gear-pinion-9 v1 (Autodesk Fusion 360 design; units mm, degrees)
description: Spur Gear; Module: 0.3; Num Teeth: 9; Pressure Angle: 20.0; Backlash: 0.00 mm
Autodesk Fusion 360 part; units mm, degrees
sketch "スケッチ1" plane through (0, 0, 0) normal (0, 0, 1) x (1, 0, 0) in component "Spur Gear (9 teeth)"
  circle A0 centre (0, 0) radius 0.9392
  circle A1 centre (0, 0) radius 0.4
extrude "押し出し1" add sketch "スケッチ1" along normal blind 1 in component "Spur Gear (9 teeth)"
sketch "スケッチ2" plane through (0, 0, 0) normal (0, 0, 1) x (1, 0, 0) in component "Spur Gear (9 teeth)"
  spline S0 degree 5 poles (1.2459, -0.2389) (1.247, -0.2391) (1.2492, -0.2395) (1.2525, -0.2399) (1.2569, -0.2403) (1.2625, -0.2405) (1.268, -0.2404) (1.2736, -0.2403) (1.2793, -0.24) (1.2849, -0.2397) (1.2906, -0.2394) (1.2962, -0.2389) (1.3019, -0.2384) (1.3076, -0.2378) (1.3134, -0.237) (1.3191, -0.2362) (1.3248, -0.2353) (1.3306, -0.2342) (1.3363, -0.2332) (1.3421, -0.232) (1.3478, -0.2308) (1.3536, -0.2295) (1.3594, -0.2282) (1.3652, -0.2268) (1.371, -0.2253) (1.3768, -0.2237) (1.3826, -0.2221) (1.3884, -0.2204) (1.3942, -0.2187) (1.4, -0.2168) (1.4058, -0.215) (1.4116, -0.213) (1.4174, -0.211) (1.4233, -0.209) (1.4291, -0.2068) (1.4349, -0.2047) (1.4407, -0.2024) (1.4466, -0.2001) (1.4524, -0.1977) (1.4582, -0.1953) (1.464, -0.1929) (1.4698, -0.1903) (1.4757, -0.1877) (1.4815, -0.1851) (1.4873, -0.1824) (1.4931, -0.1796) (1.4989, -0.1768) (1.5047, -0.1739) (1.5105, -0.171) (1.5163, -0.168) (1.5221, -0.165) (1.5279, -0.1619) (1.5337, -0.1588) (1.5394, -0.1556) (1.5452, -0.1523) (1.551, -0.149) (1.5567, -0.1457) (1.5625, -0.1423) (1.5682, -0.1388) (1.574, -0.1353) (1.5797, -0.1317) (1.5854, -0.1281) (1.5912, -0.1245) (1.5969, -0.1207) (1.6026, -0.117) (1.6083, -0.1131) (1.6139, -0.1093) (1.6196, -0.1053) (1.6253, -0.1014) (1.6309, -0.0973) (1.6366, -0.0933) (1.6411, -0.09) (1.6444, -0.0875) (1.6467, -0.0858) (1.6478, -0.085) knots 0 0 0 0 0 0 0.01428571 0.02857143 0.04285714 0.05714286 0.07142857 0.08571429 0.1 0.11428571 0.12857143 0.14285714 0.15714286 0.17142857 0.18571429 0.2 0.21428571 0.22857143 0.24285714 0.25714286 0.27142857 0.28571429 0.3 0.31428571 0.32857143 0.34285714 0.35714286 0.37142857 0.38571429 0.4 0.41428571 0.42857143 0.44285714 0.45714286 0.47142857 0.48571429 0.5 0.51428571 0.52857143 0.54285714 0.55714286 0.57142857 0.58571429 0.6 0.61428571 0.62857143 0.64285714 0.65714286 0.67142857 0.68571429 0.7 0.71428571 0.72857143 0.74285714 0.75714286 0.77142857 0.78571429 0.8 0.81428571 0.82857143 0.84285714 0.85714286 0.87142857 0.88571429 0.9 0.91428571 0.92857143 0.94285714 0.95714286 0.97142857 0.98571429 1 1 1 1 1 1
  spline S1 degree 5 poles (1.2459, 0.2389) (1.247, 0.2391) (1.2492, 0.2395) (1.2525, 0.2399) (1.2569, 0.2403) (1.2625, 0.2405) (1.268, 0.2404) (1.2736, 0.2403) (1.2793, 0.24) (1.2849, 0.2397) (1.2906, 0.2394) (1.2962, 0.2389) (1.3019, 0.2384) (1.3076, 0.2378) (1.3134, 0.237) (1.3191, 0.2362) (1.3248, 0.2353) (1.3306, 0.2342) (1.3363, 0.2332) (1.3421, 0.232) (1.3478, 0.2308) (1.3536, 0.2295) (1.3594, 0.2282) (1.3652, 0.2268) (1.371, 0.2253) (1.3768, 0.2237) (1.3826, 0.2221) (1.3884, 0.2204) (1.3942, 0.2187) (1.4, 0.2168) (1.4058, 0.215) (1.4116, 0.213) (1.4174, 0.211) (1.4233, 0.209) (1.4291, 0.2068) (1.4349, 0.2047) (1.4407, 0.2024) (1.4466, 0.2001) (1.4524, 0.1977) (1.4582, 0.1953) (1.464, 0.1929) (1.4698, 0.1903) (1.4757, 0.1877) (1.4815, 0.1851) (1.4873, 0.1824) (1.4931, 0.1796) (1.4989, 0.1768) (1.5047, 0.1739) (1.5105, 0.171) (1.5163, 0.168) (1.5221, 0.165) (1.5279, 0.1619) (1.5337, 0.1588) (1.5394, 0.1556) (1.5452, 0.1523) (1.551, 0.149) (1.5567, 0.1457) (1.5625, 0.1423) (1.5682, 0.1388) (1.574, 0.1353) (1.5797, 0.1317) (1.5854, 0.1281) (1.5912, 0.1245) (1.5969, 0.1207) (1.6026, 0.117) (1.6083, 0.1131) (1.6139, 0.1093) (1.6196, 0.1053) (1.6253, 0.1014) (1.6309, 0.0973) (1.6366, 0.0933) (1.6411, 0.09) (1.6444, 0.0875) (1.6467, 0.0858) (1.6478, 0.085) knots 0 0 0 0 0 0 0.01428571 0.02857143 0.04285714 0.05714286 0.07142857 0.08571429 0.1 0.11428571 0.12857143 0.14285714 0.15714286 0.17142857 0.18571429 0.2 0.21428571 0.22857143 0.24285714 0.25714286 0.27142857 0.28571429 0.3 0.31428571 0.32857143 0.34285714 0.35714286 0.37142857 0.38571429 0.4 0.41428571 0.42857143 0.44285714 0.45714286 0.47142857 0.48571429 0.5 0.51428571 0.52857143 0.54285714 0.55714286 0.57142857 0.58571429 0.6 0.61428571 0.62857143 0.64285714 0.65714286 0.67142857 0.68571429 0.7 0.71428571 0.72857143 0.74285714 0.75714286 0.77142857 0.78571429 0.8 0.81428571 0.82857143 0.84285714 0.85714286 0.87142857 0.88571429 0.9 0.91428571 0.92857143 0.94285714 0.95714286 0.97142857 0.98571429 1 1 1 1 1 1
  arc A0 (1.6478, -0.085) -> (1.6478, 0.085) centre (0, 0) ccw
  line L0 (0.9126, -0.1769) -> (1.2459, -0.2389)
  line L1 (0.9126, 0.1769) -> (1.2459, 0.2389)
  line L2 (0.9126, -0.1769) -> (0.9126, 0.1769)
  point P0 (1.2734, -0.2403)
  point P1 (1.3014, -0.2384)
  point P2 (1.3298, -0.2344)
  point P3 (1.3585, -0.2284)
  point P4 (1.3874, -0.2207)
  point P5 (1.4164, -0.2114)
  point P6 (1.4454, -0.2005)
  point P7 (1.4746, -0.1882)
  point P8 (1.5037, -0.1744)
  point P9 (1.5328, -0.1593)
  point P10 (1.5618, -0.1427)
  point P11 (1.5906, -0.1248)
  point P12 (1.6193, -0.1055)
  point P13 (1.2734, 0.2403)
  point P14 (1.3014, 0.2384)
  point P15 (1.3298, 0.2344)
  point P16 (1.3585, 0.2284)
  point P17 (1.3874, 0.2207)
  point P18 (1.4164, 0.2114)
  point P19 (1.4454, 0.2005)
  point P20 (1.4746, 0.1882)
  point P21 (1.5037, 0.1744)
  point P22 (1.5328, 0.1593)
  point P23 (1.5618, 0.1427)
  point P24 (1.5906, 0.1248)
  point P25 (1.6193, 0.1055)
extrude "押し出し2" add sketch "スケッチ2" along normal blind 1 in component "Spur Gear (9 teeth)"
pattern_circular "C パターン1" count 9 over 360 about axis through (0, 0, 0) along (0, 0, 1) of "押し出し2" in component "Spur Gear (9 teeth)"
sketch "スケッチ3" plane through (0, 0, 0) normal (0, 0, 1) x (1, 0, 0) in component "Spur Gear (9 teeth)"
  circle A0 centre (0, 0) radius 1.35 construction
component "Spur Gear (9 teeth)" placed x (1, 0, 0) y (0, 1, 0) z (0, 0, 1) at (0, 0, 0)
